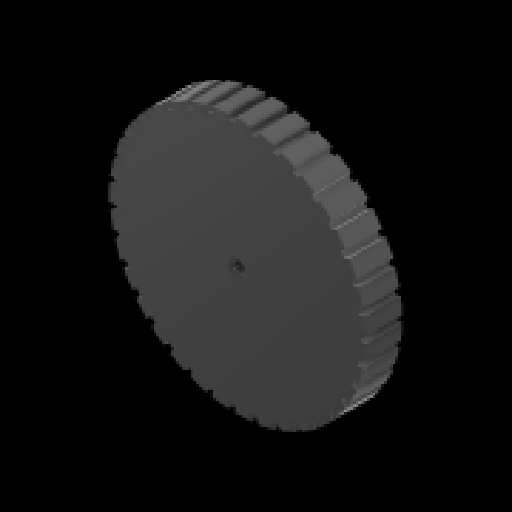
# Autodesk Inventor part: RobotWheelMK1
Saved by Autodesk Inventor 2025 (Build 290162000, 162)
## iProperties
Created: 2024-11-18
Part Number: RobotWheelMK1
Material: Generic
Document SubType Name: Modeling
Designer: Trevor
Density: 1 g/cm^3
Appearance: Default
Author: Trevor
Autodesk Inventor part; units mm, degrees
ref_plane "YZ Plane" through (0, 0, 0) normal (1, 0, 0) x (0, 1, 0)
ref_plane "XZ Plane" through (0, 0, 0) normal (0, 1, 0) x (-1, 0, 0)
ref_plane "XY Plane" through (0, 0, 0) normal (0, 0, 1) x (1, 0, 0)
sketch "Sketch1" plane through (0, 0, 0) normal (0, 0, 1) x (1, 0, 0)
  line L0 (-2.4408, -0.5408) -> (-1.2026, 2.1918) projected
  arc A0 (-2.4408, -0.5408) -> (-1.2026, 2.1918) centre (0, 0) ccw projected
  circle A1 centre (0, 0) radius 50
  line L1 (-52.2966, -3.2808) -> (-49.8922, -3.2808)
  line L2 (-49.8922, 3.2808) -> (-52.2966, 3.2808)
  line L3 (-52.2966, 3.2808) -> (-52.2966, -3.2808)
  line L4 (-52.2966, -3.2808) -> (-50, 0) construction
  line L5 (-50, 0) -> (-52.2966, 3.2808) construction
  line L6 (-49.6763, -5.6805) -> (-52.042, -6.1098)
  line L7 (-52.042, -6.1098) -> (-50.8703, -12.566)
  line L8 (-50.8703, -12.566) -> (-48.5046, -12.1367)
  circle A2 centre (0, 0) radius 50
  line L9 (-47.8637, -14.4592) -> (-50.1147, -15.3041)
  line L10 (-50.1147, -15.3041) -> (-47.8091, -21.4473)
  line L11 (-47.8091, -21.4473) -> (-45.5581, -20.6025)
  circle A3 centre (0, 0) radius 50
  line L12 (-44.5127, -22.7733) -> (-46.5767, -24.0064)
  line L13 (-46.5767, -24.0064) -> (-43.2112, -29.6393)
  line L14 (-43.2112, -29.6393) -> (-41.1472, -28.4061)
  circle A4 centre (0, 0) radius 50
  line L15 (-39.731, -30.3553) -> (-41.5417, -31.9372)
  line L16 (-41.5417, -31.9372) -> (-37.2245, -36.8787)
  line L17 (-37.2245, -36.8787) -> (-35.4138, -35.2967)
  circle A5 centre (0, 0) radius 50
  line L18 (-33.6724, -36.9618) -> (-35.1715, -38.8415)
  line L19 (-35.1715, -38.8415) -> (-30.0413, -42.9327)
  line L20 (-30.0413, -42.9327) -> (-28.5422, -41.0529)
  circle A6 centre (0, 0) radius 50
  line L21 (-26.5315, -42.3802) -> (-27.6708, -44.4975)
  line L22 (-27.6708, -44.4975) -> (-21.8926, -47.6068)
  line L23 (-21.8926, -47.6068) -> (-20.7533, -45.4896)
  circle A7 centre (0, 0) radius 50
  line L24 (-18.5378, -46.4365) -> (-19.2808, -48.7232)
  line L25 (-19.2808, -48.7232) -> (-13.0403, -50.7508)
  line L26 (-13.0403, -50.7508) -> (-12.2973, -48.4642)
  circle A8 centre (0, 0) radius 50
  line L27 (-9.9483, -49.0003) -> (-10.2711, -51.3829)
  line L28 (-10.2711, -51.3829) -> (-3.7688, -52.2637)
  line L29 (-3.7688, -52.2637) -> (-3.4461, -49.8811)
  circle A9 centre (0, 0) radius 50
  line L30 (-1.0391, -49.9892) -> (-0.9313, -52.3911)
  line L31 (-0.9313, -52.3911) -> (5.6238, -52.0967)
  line L32 (5.6238, -52.0967) -> (5.5159, -49.6948)
  circle A10 centre (0, 0) radius 50
  line L33 (7.9035, -49.3714) -> (8.4385, -51.7155)
  line L34 (8.4385, -51.7155) -> (14.8357, -50.2553)
  line L35 (14.8357, -50.2553) -> (14.3007, -47.9113)
  circle A11 centre (0, 0) radius 50
  line L36 (16.5921, -47.1668) -> (17.537, -49.3776)
  line L37 (17.537, -49.3776) -> (23.5707, -46.7987)
  line L38 (23.5707, -46.7987) -> (22.6257, -44.5879)
  circle A12 centre (0, 0) radius 50
  line L39 (24.7474, -43.4461) -> (26.0719, -45.4527)
  line L40 (26.0719, -45.4527) -> (31.5481, -41.8379)
  line L41 (31.5481, -41.8379) -> (30.2236, -39.8313)
  circle A13 centre (0, 0) radius 50
  line L42 (32.1073, -38.3291) -> (33.7688, -40.067)
  line L43 (33.7688, -40.067) -> (38.5116, -35.5324)
  line L44 (38.5116, -35.5324) -> (36.85, -33.7946)
  circle A14 centre (0, 0) radius 50
  line L45 (38.4352, -31.9802) -> (40.3804, -33.3934)
  line L46 (40.3804, -33.3934) -> (44.2373, -28.0849)
  line L47 (44.2373, -28.0849) -> (42.2921, -26.6717)
  circle A15 centre (0, 0) radius 50
  line L48 (43.5279, -24.6034) -> (45.6941, -25.6466)
  line L49 (45.6941, -25.6466) -> (48.5411, -19.7347)
  line L50 (48.5411, -19.7347) -> (46.3749, -18.6915)
  circle A16 centre (0, 0) radius 50
  line L51 (47.2214, -16.4358) -> (49.5391, -17.0754)
  line L52 (49.5391, -17.0754) -> (51.2848, -10.7502)
  line L53 (51.2848, -10.7502) -> (48.9671, -10.1106)
  circle A17 centre (0, 0) radius 50
  line L54 (49.3973, -7.7399) -> (51.792, -7.9555)
  line L55 (51.792, -7.9555) -> (52.3801, -1.4202)
  line L56 (52.3801, -1.4202) -> (49.9855, -1.2047)
  circle A18 centre (0, 0) radius 50
  line L57 (49.9855, 1.2047) -> (52.3801, 1.4202)
  line L58 (52.3801, 1.4202) -> (51.792, 7.9555)
  line L59 (51.792, 7.9555) -> (49.3973, 7.7399)
  circle A19 centre (0, 0) radius 50
  line L60 (48.9671, 10.1106) -> (51.2848, 10.7502)
  line L61 (51.2848, 10.7502) -> (49.5391, 17.0754)
  line L62 (49.5391, 17.0754) -> (47.2214, 16.4358)
  circle A20 centre (0, 0) radius 50
  line L63 (46.3749, 18.6915) -> (48.5411, 19.7347)
  line L64 (48.5411, 19.7347) -> (45.6941, 25.6466)
  line L65 (45.6941, 25.6466) -> (43.5279, 24.6034)
  circle A21 centre (0, 0) radius 50
  line L66 (42.2921, 26.6717) -> (44.2373, 28.0849)
  line L67 (44.2373, 28.0849) -> (40.3804, 33.3934)
  line L68 (40.3804, 33.3934) -> (38.4352, 31.9802)
  circle A22 centre (0, 0) radius 50
  line L69 (36.85, 33.7946) -> (38.5116, 35.5324)
  line L70 (38.5116, 35.5324) -> (33.7688, 40.067)
  line L71 (33.7688, 40.067) -> (32.1073, 38.3291)
  circle A23 centre (0, 0) radius 50
  line L72 (30.2236, 39.8313) -> (31.5481, 41.8379)
  line L73 (31.5481, 41.8379) -> (26.0719, 45.4527)
  line L74 (26.0719, 45.4527) -> (24.7474, 43.4461)
  circle A24 centre (0, 0) radius 50
  line L75 (22.6257, 44.5879) -> (23.5707, 46.7987)
  line L76 (23.5707, 46.7987) -> (17.537, 49.3776)
  line L77 (17.537, 49.3776) -> (16.5921, 47.1668)
  circle A25 centre (0, 0) radius 50
  line L78 (14.3007, 47.9113) -> (14.8357, 50.2553)
  line L79 (14.8357, 50.2553) -> (8.4385, 51.7155)
  line L80 (8.4385, 51.7155) -> (7.9035, 49.3714)
  circle A26 centre (0, 0) radius 50
  line L81 (5.5159, 49.6948) -> (5.6238, 52.0967)
  line L82 (5.6238, 52.0967) -> (-0.9313, 52.3911)
  line L83 (-0.9313, 52.3911) -> (-1.0391, 49.9892)
  circle A27 centre (0, 0) radius 50
  line L84 (-3.4461, 49.8811) -> (-3.7688, 52.2637)
  line L85 (-3.7688, 52.2637) -> (-10.2711, 51.3829)
  line L86 (-10.2711, 51.3829) -> (-9.9483, 49.0003)
  circle A28 centre (0, 0) radius 50
  line L87 (-12.2973, 48.4642) -> (-13.0403, 50.7508)
  line L88 (-13.0403, 50.7508) -> (-19.2808, 48.7232)
  line L89 (-19.2808, 48.7232) -> (-18.5378, 46.4365)
  circle A29 centre (0, 0) radius 50
  line L90 (-20.7533, 45.4896) -> (-21.8926, 47.6068)
  line L91 (-21.8926, 47.6068) -> (-27.6708, 44.4975)
  line L92 (-27.6708, 44.4975) -> (-26.5315, 42.3802)
  circle A30 centre (0, 0) radius 50
  line L93 (-28.5422, 41.0529) -> (-30.0413, 42.9327)
  line L94 (-30.0413, 42.9327) -> (-35.1715, 38.8415)
  line L95 (-35.1715, 38.8415) -> (-33.6724, 36.9618)
  circle A31 centre (0, 0) radius 50
  line L96 (-35.4138, 35.2967) -> (-37.2245, 36.8787)
  line L97 (-37.2245, 36.8787) -> (-41.5417, 31.9372)
  line L98 (-41.5417, 31.9372) -> (-39.731, 30.3553)
  circle A32 centre (0, 0) radius 50
  line L99 (-41.1472, 28.4061) -> (-43.2112, 29.6393)
  line L100 (-43.2112, 29.6393) -> (-46.5767, 24.0064)
  line L101 (-46.5767, 24.0064) -> (-44.5127, 22.7733)
  circle A33 centre (0, 0) radius 50
  line L102 (-45.5581, 20.6025) -> (-47.8091, 21.4473)
  line L103 (-47.8091, 21.4473) -> (-50.1147, 15.3041)
  line L104 (-50.1147, 15.3041) -> (-47.8637, 14.4592)
  circle A34 centre (0, 0) radius 50
  line L105 (-48.5046, 12.1367) -> (-50.8703, 12.566)
  line L106 (-50.8703, 12.566) -> (-52.042, 6.1098)
  line L107 (-52.042, 6.1098) -> (-49.6763, 5.6805)
  circle A35 centre (0, 0) radius 50
  point P0 (0, 0)
  point P1 (-49.1965, -8.9278)
  point P2 (-46.8117, -17.5687)
  point P3 (-42.9224, -25.645)
  point P4 (-37.6536, -32.8969)
  point P5 (-31.1745, -39.0916)
  point P6 (-23.6934, -44.0298)
  point P7 (-15.4508, -47.5528)
  point P8 (-6.7117, -49.5475)
  point P9 (2.2432, -49.9497)
  point P10 (11.126, -48.7464)
  point P11 (19.6513, -45.9764)
  point P12 (27.5448, -41.7287)
  point P13 (34.5531, -36.1397)
  point P14 (40.4508, -29.3893)
  point P15 (45.0484, -21.6942)
  point P16 (48.1981, -13.3018)
  point P17 (49.7987, -4.482)
  point P18 (49.7987, 4.482)
  point P19 (48.1981, 13.3018)
  point P20 (45.0484, 21.6942)
  point P21 (40.4508, 29.3893)
  point P22 (34.5531, 36.1397)
  point P23 (27.5448, 41.7287)
  point P24 (19.6513, 45.9764)
  point P25 (11.126, 48.7464)
  point P26 (2.2432, 49.9497)
  point P27 (-6.7117, 49.5475)
  point P28 (-15.4508, 47.5528)
  point P29 (-23.6934, 44.0298)
  point P30 (-31.1745, 39.0916)
  point P31 (-37.6536, 32.8969)
  point P32 (-42.9224, 25.645)
  point P33 (-46.8117, 17.5687)
  point P34 (-49.1965, 8.9278)
  dimension "d0" = 100
  dimension "d5" = 360
  constraints: 214 end point, 102 point on circle, 34 centre point, 2 coincident with centre, 1 coincident, 1 horizontal, 1 parallel, 354 other
ref_plane "Work Plane1" through (-2, -2, 15) normal (0, 0, 1) x (1, 0, 0)
extrude "Extrusion1" add sketch "Sketch1" along normal up to surface (15 mm away)
body "Solid1"
